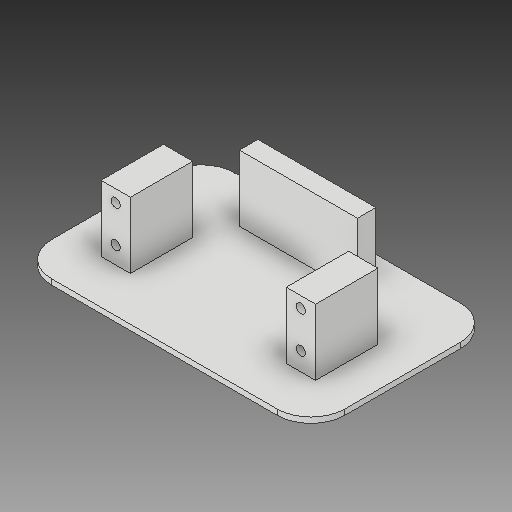
# Autodesk Inventor part: capaservo
Saved by Autodesk Inventor 2017 (Build 210142000, 142)
## iProperties
Created: 2017-12-20
Part Number: capaservo
Material: Generic
Document SubType Name: Modeling
Designer: will
Density: 1 g/cm^3
Appearance: Default
Author: will
Autodesk Inventor part; units mm, degrees
ref_plane "YZ Plane" through (0, 0, 0) normal (1, 0, 0) x (0, 1, 0)
ref_plane "XZ Plane" through (0, 0, 0) normal (0, 1, 0) x (-1, 0, 0)
ref_plane "XY Plane" through (0, 0, 0) normal (0, 0, 1) x (1, 0, 0)
sketch "Sketch1" plane through (0, 0, 0) normal (0, 1, 0) x (-1, 0, 0)
  line L0 (10.7789, 2.112) -> (-69.2211, 2.112)
  line L1 (-69.2211, 2.112) -> (-69.2211, -47.888)
  line L2 (-69.2211, -47.888) -> (10.7789, -47.888)
  line L3 (10.7789, -47.888) -> (10.7789, 2.112)
  line L4 (-2.3383, -18.388) -> (10.7789, -18.388) construction
  dimension "d0" = 80
  dimension "d1" = 50
  constraints: 10 end point, 2 parallel, 2 perpendicular, 1 horizontal, 1 point on line
  measures "d0" distance of L2.end L1.end
  measures "d1" distance of L1.end L0.end
sketch "Sketch2" plane through (0, 0, 0) normal (0, 1, 0) x (-1, 0, 0)
  line L0 (10.7789, 2.112) -> (-69.2211, 2.112)
  line L1 (-69.2211, 2.112) -> (-69.2211, -47.888)
  line L2 (-69.2211, -47.888) -> (10.7789, -47.888)
  line L3 (10.7789, -47.888) -> (10.7789, 2.112)
  line L4 (-7.9711, -9.888) -> (0.0289, -9.888)
  line L5 (0.0289, -9.888) -> (0.0289, -26.888)
  line L6 (0.0289, -26.888) -> (-7.9711, -26.888)
  line L7 (-7.9711, -26.888) -> (-7.9711, -9.888)
  line L8 (-58.4711, -9.888) -> (-50.4711, -9.888)
  line L9 (-50.4711, -9.888) -> (-50.4711, -26.888)
  line L10 (-50.4711, -26.888) -> (-58.4711, -26.888)
  line L11 (-58.4711, -26.888) -> (-58.4711, -9.888)
  line L12 (0.0289, -18.388) -> (10.7789, -18.388) construction
  line L13 (-58.4711, -18.388) -> (-69.2211, -18.388) construction
  line L14 (-11.702, -35.888) -> (-43.8801, -35.888)
  line L15 (-43.8801, -35.888) -> (-43.8801, -40.926)
  line L16 (-43.8801, -40.926) -> (-11.702, -40.926)
  line L17 (-11.702, -40.926) -> (-11.702, -35.888)
  point P0 (0, 0)
  point P1 (0, 0)
  dimension "d6" = 80
  dimension "d7" = 50
  dimension "d8" = 42.5
  dimension "d9" = 12
  dimension "d10" = 17
  dimension "d11" = 38
  dimension "d16" = 8
  constraints: 36 end point, 8 parallel, 5 perpendicular, 5 point on line, 4 horizontal, 2 collinear, 2 midpoint
  measures "d6" distance of L2.end L2.start
  measures "d7" distance of L2.start L0.end
  measures "d8" distance between parallel lines of L9 L7
  measures "d9" distance between parallel lines of L0 L4
  measures "d10" distance of L4.end L5.end
  measures "d11" distance between parallel lines of L0 L14
  measures "d16" distance of L8.start L9.start
extrude "Extrusion1" add sketch "Sketch1" against normal blind 1.5
extrude "Extrusion2" add sketch "Sketch2" along normal blind 18 contours L4 L5 L6 L7 | L8 L9 L10 L11 | L17 L16 L15 L14
sketch "Sketch3" plane through (-0.0289, 0, -9.888) normal (0, 0, 1) x (1, 0, 0)
  line L0 (8, 0) -> (0, 0) projected
  line L1 (8, 0) -> (8, 18) projected
  line L2 (0, 18) -> (8, 18) projected
  line L3 (0, 0) -> (0, 18) projected
  line L4 (58.5, 0) -> (50.5, 0) projected
  line L5 (58.5, 0) -> (58.5, 18) projected
  line L6 (50.5, 18) -> (58.5, 18) projected
  line L7 (50.5, 0) -> (50.5, 18) projected
  circle A0 centre (54.5, 5) radius 1.25
  circle A1 centre (4, 4.6892) radius 1.25
  circle A2 centre (54.5, 15) radius 1.25
  circle A3 centre (4, 14.6892) radius 1.25
  point P0 (0.0289, 0)
  dimension "d17" = 5
  dimension "d18" = 10
  dimension "d19" = 10
  dimension "d20" = 2.5
  constraints: 4 centre point, 3 equal radius
  measures "d17" distance from line of L4 A0.centre
  measures "d18" distance of A0.centre A2.centre
  measures "d19" distance of A1.centre A3.centre
  measures "d20" diameter of A1
extrude "Extrusion3" cut sketch "Sketch3" against normal blind 4.5 contours A0 | A1 | A2 | A3
fillet "Fillet1" radius 9.25 4 edges at (69.2211, -0.75, 2.112) (-10.7789, -0.75, 2.112) (-10.7789, -0.75, -47.888) (69.2211, -0.75, -47.888)
body "Solid1"
